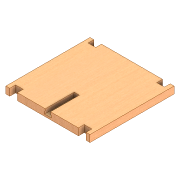
# Autodesk Inventor part: TNS-1-platform
Saved by Autodesk Inventor 2020 (Build 240168000, 168)
## iProperties
Created: 2021-06-28
Part Number: TNS-1-platform
Material: Generic
Document SubType Name: Modeling
Designer: Aidan Lee
Density: 1 g/cm^3
Appearance: Cherry - Natural Low Gloss
Author: Aidan Lee
Autodesk Inventor part; units mm, degrees
ref_plane "YZ Plane" through (0, 0, 0) normal (1, 0, 0) x (0, 1, 0)
ref_plane "XZ Plane" through (0, 0, 0) normal (0, 1, 0) x (-1, 0, 0)
ref_plane "XY Plane" through (0, 0, 0) normal (0, 0, 1) x (1, 0, 0)
sketch "Sketch1" plane through (0, 0, 0) normal (0, 0, 1) x (1, 0, 0)
  line L0 (0, 0) -> (219, 0)
  line L1 (219, 0) -> (219, 18)
  line L2 (219, 18) -> (0, 18)
  line L3 (0, 18) -> (0, 0)
  dimension "d0" = 219
  dimension "d1" = 18
  constraints: 8 end point, 2 parallel, 1 horizontal, 1 perpendicular
  measures "d0" distance of L0.start L0.end
  measures "d1" distance of L2.end L0.start
extrude "Extrusion1" add sketch "Sketch1" along normal blind 219
sketch "Sketch2" plane through (0, 0, 219) normal (0, 0, 1) x (1, 0, 0)
  line L0 (102.6988, 18) -> (100.5, 5)
  line L1 (100.5, 5) -> (118.5, 5)
  line L2 (0, 0) -> (219, 0) projected
  line L3 (219, 18) -> (0, 18) projected
  line L4 (102.6988, 18) -> (102.6988, 9.1069) construction
  line L5 (109.5, -2.3259) -> (109.5, -4.6671) construction
  line L6 (116.3012, 18) -> (118.5, 5)
  point P0 (109.5, 5)
  point P1 (109.5, 0)
  point P2 (109.5, -3.4965)
  point P3 (109.5, 0)
  dimension "d4" = 5
  dimension "d5" = 9.6
  dimension "d6" = 18
  constraints: 10 end point, 4 midpoint, 2 vertical, 2 vertical alignment, 1 horizontal, 1 point on line, 1 symmetric about line
  measures "d4" distance between parallel lines of L2 L1
  measures "d5" angle of L4 L0
  measures "d6" distance of L0.end L1.end
extrude "Extrusion2" cut sketch "Sketch2" against normal blind 75
sketch "Sketch3" plane through (0, 18, 0) normal (0, 1, 0) x (1, 0, 0)
  line L0 (10, -204) -> (30, -204)
  line L1 (0, 0) -> (0, -219) projected
  line L2 (20, -205.0009) -> (20, -197.8859) construction
  line L3 (102.6988, -219) -> (0, -219) construction
  line L4 (10, -204) -> (10, -219)
  line L5 (30, -204) -> (30, -219)
  line L6 (30, -219) -> (10, -219)
  point P0 (20, -204)
  dimension "d17" = 20
  dimension "d18" = 15
  dimension "d19" = 10
  constraints: 10 end point, 2 point on line, 2 vertical, 1 collinear, 1 horizontal, 1 midpoint, 1 perpendicular, 1 vertical alignment
  measures "d17" distance of L0.start L0.end
  measures "d18" distance between parallel lines of L3 L0
  measures "d19" distance between parallel lines of L1 L4
extrude "Extrusion3" cut sketch "Sketch3" against normal through all
pattern_linear "Rectangular Pattern1" count 2 spacing -204 along (0, 0, 1) count 2 spacing 179 along (1, 0, 0) of "Extrusion3"
body "Solid1"
